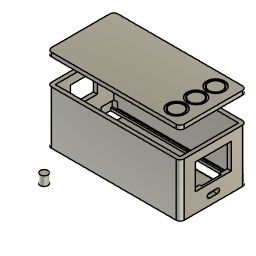
SmartClock v7 (Autodesk Fusion 360 design; units mm, degrees)
Autodesk Fusion 360 part; units mm, degrees
sketch "Sketch1" plane through (0, 0, 0) normal (0, 0, 1) x (1, 0, 0)
  line L0 (0, 0) -> (100, 0)
  line L1 (100, 0) -> (100, 50)
  line L2 (100, 50) -> (0, 50)
  line L3 (0, 50) -> (0, 0)
  line L4 (97, 47) -> (3, 47)
  line L5 (3, 47) -> (3, 3)
  line L6 (3, 3) -> (97, 3)
  line L7 (97, 3) -> (97, 47)
  dimension "boxOuterWidth" = 100
  dimension "boxOuterLength" = 50
  dimension "d3" = -3
  constraint horizontal L0
  constraint vertical L1
  constraint horizontal L2
  constraint vertical L3
  constraint coincident L0.start L3.end
  measures "boxOuterWidth" distance of L0.start L0.end
  measures "boxOuterLength" distance of L0.start L2.end
extrude "Extrude1" add sketch "Sketch1" along normal blind 3 contours L4 L5 L6 L7 makes body 1
extrude "Extrude2" add sketch "Sketch1" along normal blind 40 bodies 1
sketch "Sketch2" plane through (0, 0, 0) normal (-1, 0, 0) x (0, -1, 0)
  line L0 (-50, 0) -> (0, 0)
  line L1 (0, 0) -> (0, 40)
  line L2 (0, 40) -> (-50, 40)
  line L3 (-50, 40) -> (-50, 0)
  line L4 (-3, 3) -> (-47, 3)
  line L5 (-47, 3) -> (-47, 40)
  line L6 (-47, 40) -> (-3, 40)
  line L7 (-3, 40) -> (-3, 3)
  line L8 (-27.975, 12.2) -> (-22.025, 12.2)
  line L9 (-27.975, 8.7) -> (-22.025, 8.7)
  arc A0 (-22.025, 8.7) -> (-22.025, 12.2) centre (-22.025, 10.45) ccw
  arc A1 (-27.975, 12.2) -> (-27.975, 8.7) centre (-27.975, 10.45) ccw
  line L10 (-34.65, 34) -> (-34.65, 17.9)
  line L11 (-34.65, 17.9) -> (-14.35, 17.9)
  line L12 (-14.35, 17.9) -> (-14.35, 34)
  line L13 (-14.35, 34) -> (-34.65, 34)
  circle A2 centre (-12.1, 25.95) radius 1.4
  line L14 (-14.35, 25.95) -> (-34.65, 25.95) construction
  line L15 (-14.35, 25.95) -> (-12.1, 25.95) construction
  circle A3 centre (-12.1, 25.95) radius 2.25
  line L16 (-34.65, 25.95) -> (-39.95, 25.95) construction
  circle A4 centre (-39.95, 25.95) radius 1.45
  circle A5 centre (-39.95, 25.95) radius 2.5
  dimension "d8" = 5.95
  dimension "d9" = 3.5
  dimension "d10" = 16.1
  dimension "d11" = 20.3
  dimension "d12" = 2.8
  dimension "d13" = 2.25
  dimension "d19" = 5.3
  dimension "d20" = 2.9
  dimension "d21" = 5
  dimension "d25" = 12.35
  dimension "d26" = 6
  dimension "d27" = 5.7
  dimension "d28" = 5.7
  dimension "d29" = 19.025
  dimension "d30" = 19.025
  constraint horizontal L8
  constraint parallel L8 L9
  constraint tangent L9 A0
  constraint tangent L8 A0
  constraint tangent L9 A1
  constraint tangent L8 A1
  constraint midpoint L12 L14.start
  constraint midpoint L10 L14.end
  constraint perpendicular L12 L15
  constraint coincident A2.centre L15.end
  constraint concentric A2 A3
  constraint coincident L14.start A3
  constraint coincident L16.end A4.centre
  constraint perpendicular L10 L11
  constraint perpendicular L11 L12
  constraint perpendicular L12 L13
  constraint collinear L14 L16
  measures "d8" distance of L8.start L8.end
  measures "d9" distance of L8 L9
  measures "d10" distance of L10.start L10.end
  measures "d11" distance of L10.start L12.end
  measures "d12" diameter of A2
  measures "d13" distance of L12 A2.centre
  measures "d19" distance of L14.end L16.end
  measures "d20" diameter of A4
  measures "d21" diameter of A5
  measures "d25" distance of L5 L10
  measures "d26" distance of L2 L13
  measures "d27" distance of L4 L9
  measures "d28" distance of L8 L11
  measures "d29" distance of L5 A1.centre
  measures "d30" distance of L7 A0.centre
extrude "Extrude3" cut sketch "Sketch2" against normal up to surface (3 mm away) contours L8 L9 A0 A1 | L10 L11 L12 L13 bodies 1
extrude "Extrude4" add sketch "Sketch2" against normal blind 2 from surface at -3 contours A3 bodies 1
extrude "Extrude5" add sketch "Sketch2" against normal blind 4 from surface at -3 contours A5 bodies 1
sketch "Sketch3" plane through (100, 0, 0) normal (1, 0, 0) x (0, 1, 0)
  line L0 (0, 0) -> (50, 0)
  line L1 (50, 0) -> (50, 40)
  line L2 (50, 40) -> (0, 40)
  line L3 (0, 40) -> (0, 0)
  line L4 (47, 3) -> (3, 3)
  line L5 (3, 3) -> (3, 40)
  line L6 (3, 40) -> (47, 40)
  line L7 (47, 40) -> (47, 3)
  line L8 (22.025, 8.35) -> (27.975, 8.35)
  line L9 (22.025, 4.85) -> (27.975, 4.85)
  arc A0 (27.975, 4.85) -> (27.975, 8.35) centre (27.975, 6.6) ccw
  arc A1 (22.025, 8.35) -> (22.025, 4.85) centre (22.025, 6.6) ccw
  line L10 (19.5, 34.5) -> (30.5, 34.5)
  line L11 (13.25, 36) -> (36.75, 12.2) construction
  line L12 (38.55, 33.73) -> (38.55, 14.33)
  line L13 (13.25, 12.2) -> (13.25, 36) construction
  line L14 (36.75, 36) -> (36.75, 12.2) construction
  circle A2 centre (36.75, 36) radius 1.375
  line L15 (11.25, 33.73) -> (11.45, 33.73) construction
  line L16 (13.128, 19.766) -> (36.872, 19.766)
  line L17 (11.25, 38) -> (11.25, 33.73) construction
  line L18 (30.5, 38) -> (19.5, 38)
  line L19 (38.75, 32.63) -> (36.872, 32.63) construction
  line L20 (11.45, 33.73) -> (38.55, 33.73)
  line L21 (30.5, 34.5) -> (30.5, 38)
  line L22 (38.75, 38) -> (11.25, 38)
  circle A3 centre (36.75, 36) radius 0.975
  line L23 (19.5, 38) -> (19.5, 34.5)
  circle A4 centre (36.75, 12.2) radius 1.375
  circle A5 centre (13.25, 36) radius 0.975
  line L24 (17.5, 10.2) -> (17.5, 14.2)
  line L25 (13.128, 32.63) -> (13.128, 19.766)
  circle A6 centre (13.25, 36) radius 1.375
  line L26 (11.45, 14.33) -> (11.45, 33.73)
  line L27 (32.5, 14.2) -> (32.5, 14.33)
  line L28 (36.872, 32.63) -> (13.128, 32.63)
  line L29 (32.5, 10.2) -> (17.5, 14.2) construction
  line L30 (36.872, 19.766) -> (36.872, 32.63)
  circle A7 centre (13.25, 12.2) radius 0.975
  line L31 (38.75, 38) -> (38.75, 32.63) construction
  line L32 (13.25, 36) -> (36.75, 36) construction
  line L33 (38.55, 14.33) -> (11.45, 14.33)
  circle A8 centre (36.75, 12.2) radius 0.975
  line L34 (32.5, 10.2) -> (17.5, 10.2)
  circle A9 centre (13.25, 12.2) radius 1.375
  line L35 (17.5, 10.2) -> (32.5, 14.2) construction
  line L36 (17.5, 14.2) -> (17.5, 14.33)
  line L37 (36.75, 12.2) -> (13.25, 12.2) construction
  line L38 (17.5, 14.2) -> (32.5, 14.2)
  line L39 (11.25, 10.2) -> (38.75, 10.2)
  line L40 (32.5, 14.2) -> (32.5, 10.2)
  line L41 (38.75, 10.2) -> (38.75, 38)
  line L42 (11.25, 38) -> (38.75, 10.2) construction
  line L43 (11.25, 38) -> (11.25, 10.2)
  line L44 (25, 38) -> (30.5, 38) construction
  line L45 (38.75, 38) -> (11.25, 10.2) construction
  line L46 (36.75, 36) -> (13.25, 12.2) construction
  line L47 (25, 40) -> (25, 3) construction
  line L48 (17.5, 14.2) -> (17.5, 14.33)
  line L49 (32.5, 14.2) -> (32.5, 14.33)
  point P0 (25, 12.2)
  point P1 (25, 24.1)
  point P2 (25, 24.1)
  dimension "d31" = 3.5
  dimension "d32" = 5.95
  dimension "d33" = 27.5
  dimension "d34" = 27.8
  dimension "d35" = 23.5
  dimension "d36" = 23.8
  dimension "d37" = 1.95
  dimension "d38" = 1.95
  dimension "d39" = 1.95
  dimension "d40" = 1.95
  dimension "d41" = 5.37
  dimension "d42" = 1.878
  dimension "d43" = 23.744
  dimension "d44" = 12.864
  dimension "d45" = 4.27
  dimension "d46" = 0.2
  dimension "d47" = 27.1
  dimension "d48" = 19.4
  dimension "d49" = 5.5
  dimension "d50" = 11
  dimension "d51" = 3.5
  dimension "d52" = 15
  dimension "d53" = 2.75
  dimension "d54" = 2.75
  dimension "d55" = 2.75
  dimension "d56" = 2.75
  dimension "d57" = 19.025
  dimension "d58" = 19.025
  dimension "d59" = 2
  dimension "d60" = 1.85
  dimension "d61" = 1.85
  constraint perpendicular L3 L8
  constraint parallel L8 L9
  constraint tangent L9 A0
  constraint tangent L8 A0
  constraint tangent L9 A1
  constraint tangent L8 A1
  constraint horizontal L22
  constraint perpendicular L22 L43
  constraint parallel L22 L39
  constraint parallel L41 L43
  constraint coincident P2 L45
  constraint coincident P2 L42
  constraint horizontal L32
  constraint perpendicular L14 L32
  constraint parallel L32 L37
  constraint parallel L13 L14
  constraint coincident P2 L11
  constraint coincident P2 L46
  constraint coincident P2 P1
  constraint coincident L11.start L13.end
  constraint perpendicular L22 L31
  constraint perpendicular L19 L31
  constraint horizontal L28
  constraint vertical L25
  constraint horizontal L16
  constraint vertical L30
  constraint perpendicular L17 L22
  constraint perpendicular L15 L17
  constraint horizontal L20
  constraint vertical L12
  constraint horizontal L33
  constraint vertical L26
  constraint midpoint L44.start L22
  constraint horizontal L18
  constraint vertical L23
  constraint horizontal L10
  constraint vertical L21
  constraint horizontal L34
  constraint perpendicular L24 L34
  constraint parallel L34 L38
  constraint parallel L24 L40
  constraint coincident P0 L29
  constraint coincident P0 L35
  constraint coincident L29.start L39
  constraint midpoint P0 L37
  constraint coincident L36.end L33
  constraint perpendicular L33 L36
  constraint coincident L27.end L33
  constraint perpendicular L27 L33
  constraint concentric A2 A3
  constraint concentric A4 A8
  constraint concentric A7 A9
  constraint concentric A5 A6
  constraint midpoint L6 L47.start
  constraint midpoint L4 L47.end
  constraint coincident P2 L47
  constraint coincident L18.start L22
  constraint coincident L14.start A2.centre
  constraint coincident L11.end L14.end
  constraint coincident L13.start A7.centre
  measures "d31" distance of L8 L9
  measures "d32" distance of L8.start L8.end
  measures "d33" distance of L39.start L39.end
  measures "d34" distance of L39.start L17.start
  measures "d35" distance of L11.end L13.start
  measures "d36" distance of L11.end L14.start
  measures "d37" diameter of A5
  measures "d38" diameter of A7
  measures "d39" diameter of A8
  measures "d40" diameter of A3
  measures "d41" distance of L22.start L19.start
  measures "d42" distance of L19.start L19.end
  measures "d43" distance of L25.start L19.end
  measures "d44" distance of L19.end L16.end
  measures "d45" distance of L15.start L17.start
  measures "d46" distance of L15.start L15.end
  measures "d47" distance of L12.start L15.end
  measures "d48" distance of L26.start L15.end
  measures "d49" distance of L18.start L44.start
  measures "d50" distance of L18.start L18.end
  measures "d51" distance of L18.start L10.end
  measures "d52" distance of L27.start L24.end
  measures "d53" diameter of A2
  measures "d54" diameter of A4
  measures "d55" diameter of A9
  measures "d56" diameter of A6
  measures "d57" distance of L5 A1.centre
  measures "d58" distance of L7 A0.centre
  measures "d59" distance of L2 L22
  measures "d60" distance of L8 L39
  measures "d61" distance of L4 L9
extrude "Extrude6" cut sketch "Sketch3" against normal up to surface (3 mm away) contours L8 L9 A0 A1 | L12 L20 L26 L33 | L16 L25 L28 L30 bodies 1
extrude "Extrude7" cut sketch "Sketch3" along normal blind 2 from surface at -3 contours A3 | A5 | A7 | A8 bodies 1
extrude "Extrude8" add sketch "Sketch3" against normal blind 0.5 from surface at -3 contours A2 | A4 | A6 | A9 bodies 1
extrude "Extrude9" cut sketch "Sketch3" along normal blind 1.5 from surface at -3 contours L24 L34 L38 L39 L40 | L27 L33 L36 L38 L48 L49 bodies 1
fillet "Fillet1" radius 3 4 edges at (0, 0, 20) (0, 50, 20) (100, 50, 20) (100, 0, 20) on bodies 1
extrude "Extrude10" add 1 faces at (34.3333, 17.6667, 3) along direction (0, 0, 1) blind 3 from surface at 37 separate body on bodies 1 makes body 2
extrude "Extrude11" add 1 faces at (65.6667, 1, 40) along direction (0, 0, 1) blind 3 separate body on bodies 1 makes body 3
move_body "Move1" bodies 2 3 to x (1, 0, 0) y (0, 1, 0) z (0, 0, 1) at (0, 0, 19.6311)
extrude "Extrude12" add 1 faces at (34.3333, 17.6667, 59.6311) along direction (0, 0, -1) blind 2 on bodies 2 bodies 2 3
sketch "Sketch4" plane through (0, 0, 57.6311) normal (0, 0, -1) x (1, 0, 0)
  line L0 (97, -3) -> (3, -3)
  line L1 (3, -3) -> (3, -47)
  line L2 (3, -47) -> (97, -47)
  line L3 (97, -47) -> (97, -3)
  line L4 (87, -3) -> (87, -47) construction
  circle A0 centre (87, -39.6667) radius 5
  circle A1 centre (87, -25) radius 5
  circle A2 centre (87, -10.3333) radius 5
  circle A3 centre (87, -10.3333) radius 6.75
  circle A4 centre (87, -25) radius 6.75
  circle A5 centre (87, -39.6667) radius 6.75
  circle A6 centre (87, -39.6667) radius 5.5
  circle A7 centre (87, -25) radius 5.5
  circle A8 centre (87, -10.3333) radius 5.5
  dimension "d82" = 10
  dimension "d83" = 10
  dimension "d84" = 10
  dimension "d85" = 10
  dimension "d86" = 7.3333
  dimension "d87" = 14.6667
  dimension "d88" = 14.6667
  dimension "d90" = 7.3333
  dimension "d91" = 1.75
  dimension "d92" = 1.75
  dimension "d93" = 1.75
  dimension "d99" = 0.5
  dimension "d100" = 0.5
  dimension "d101" = 0.5
  constraint coincident L0 L4.start
  constraint coincident L2 L4.end
  constraint perpendicular L2 L4
  constraint coincident L4 A0.centre
  constraint coincident L4 A1.centre
  constraint coincident L4 A2.centre
  measures "d82" distance of L3 L4
  measures "d83" diameter of A0
  measures "d84" diameter of A1
  measures "d85" diameter of A2
  measures "d86" distance of L2 A0.centre
  measures "d87" distance of A0.centre A1.centre
  measures "d88" distance of A1.centre A2.centre
  measures "d90" distance of L0 A2.centre
extrude "Extrude13" cut sketch "Sketch4" against normal blind 4.6 contours A0 | A1 | A2 bodies 2
extrude "Extrude14" cut sketch "Sketch4" along normal blind 0.5 from surface at -5 contours A3 | A4 | A5 bodies 2
sketch "Sketch5" plane through (0, 0, 0) normal (0, 0, -1) x (1, 0, 0)
  arc A0 (100, -3) -> (97, 0) centre (97, -3) ccw
  line L0 (0, -3) -> (0, -47)
  arc A1 (0, -47) -> (3, -50) centre (3, -47) ccw
  line L1 (3, -50) -> (97, -50)
  arc A2 (97, -50) -> (100, -47) centre (97, -47) ccw
  line L2 (100, -47) -> (100, -3)
  line L3 (0.8, -2) -> (99.2, -2)
  line L4 (99.2, -2) -> (99.2, -12.5)
  line L5 (99.2, -12.5) -> (0.8, -12.5)
  line L6 (0.8, -12.5) -> (0.8, -2)
  arc A3 (100, -3) -> (97, 0) centre (97, -3) ccw
  line L7 (99.2, -48) -> (0.8, -48)
  line L8 (0.8, -48) -> (0.8, -37.5)
  line L9 (0.8, -37.5) -> (99.2, -37.5)
  line L10 (99.2, -37.5) -> (99.2, -48)
  line L11 (3, 0) -> (97, 0)
  line L12 (99.2, -42.75) -> (0.8, -42.75) construction
  line L13 (0.8, -46.75) -> (99.2, -46.75)
  line L14 (99.2, -46.75) -> (99.2, -38.75)
  line L15 (99.2, -38.75) -> (0.8, -38.75)
  line L16 (0.8, -38.75) -> (0.8, -46.75)
  line L17 (0.8, -46.75) -> (99.2, -38.75) construction
  line L18 (99.2, -46.75) -> (0.8, -38.75) construction
  line L19 (0.8, -7.25) -> (99.2, -7.25) construction
  line L20 (99.2, -3.25) -> (0.8, -3.25)
  line L21 (0.8, -3.25) -> (0.8, -11.25)
  line L22 (0.8, -11.25) -> (99.2, -11.25)
  line L23 (99.2, -11.25) -> (99.2, -3.25)
  line L24 (99.2, -3.25) -> (0.8, -11.25) construction
  line L25 (0.8, -3.25) -> (99.2, -11.25) construction
  line L26 (5.8, -48) -> (5.8, -2)
  line L27 (94.2, -2) -> (94.2, -48)
  circle A4 centre (8.8, -15.5) radius 3
  circle A5 centre (91.2, -15.5) radius 3
  circle A6 centre (91.2, -34.5) radius 3
  circle A7 centre (8.8, -34.5) radius 3
  point P0 (50, -42.75)
  point P1 (50, -7.25)
  dimension "d102" = 98.4
  dimension "d103" = 10.5
  dimension "d106" = 98.4
  dimension "d107" = 10.5
  dimension "d111" = 2
  dimension "d112" = 0.8
  dimension "d113" = 0.8
  dimension "d114" = 2
  dimension "d115" = 0.8
  dimension "d124" = 8
  dimension "d127" = 8
  dimension "d128" = 5
  dimension "d132" = 5
  dimension "d133" = 3
  dimension "d134" = 3
  dimension "d135" = 3
  dimension "d136" = 3
  constraint horizontal L3
  constraint vertical L4
  constraint horizontal L5
  constraint vertical L6
  constraint horizontal L9
  constraint vertical L10
  constraint horizontal L7
  constraint vertical L8
  constraint midpoint L10 L12.start
  constraint midpoint L8 L12.end
  constraint horizontal L13
  constraint perpendicular L13 L14
  constraint parallel L13 L15
  constraint parallel L14 L16
  constraint coincident L17 P0
  constraint coincident L18 P0
  constraint coincident L8 L13.start
  constraint midpoint L12 P0
  constraint midpoint L6 L19.start
  constraint midpoint L4 L19.end
  constraint horizontal L20
  constraint perpendicular L20 L21
  constraint parallel L20 L22
  constraint parallel L21 L23
  constraint coincident L24 P1
  constraint coincident L25 P1
  constraint coincident L4 L20.start
  constraint midpoint L19 P1
  constraint coincident L7 L26.start
  constraint coincident L3 L26.end
  constraint perpendicular L3 L26
  constraint coincident L3 L27.start
  constraint coincident L7 L27.end
  constraint perpendicular L7 L27
  constraint tangent L5 A4
  constraint tangent L26 A4
  constraint tangent L5 A5
  constraint tangent L27 A5
  constraint tangent L9 A6
  constraint tangent L27 A6
  constraint tangent L26 A7
  constraint tangent L9 A7
  measures "d102" distance of L3.start L3.end
  measures "d103" distance of L3.start L5.end
  measures "d106" distance of L9.end L8.end
  measures "d107" distance of L7.end L8.end
  measures "d111" distance of L3 L11
  measures "d112" distance of L0 L6
  measures "d113" distance of L2 L4
  measures "d114" distance of L1 L7
  measures "d115" distance of L0 L8
  measures "d124" distance of L13.end L14.end
  measures "d127" distance of L20.end L21.end
  measures "d128" distance of L8 L26
  measures "d132" distance of L10 L27
  measures "d133" radius of A4
  measures "d134" radius of A5
  measures "d135" radius of A6
  measures "d136" radius of A7
extrude "Extrude15" cut sketch "Sketch5" along normal blind 1 and the other way blind 1 from surface at -3 contours L3 L6 L20 L26 | L3 L20 L26 L27 | L6 L20 L21 L22 L26 | L3 L4 L20 L27 | L20 L22 L26 L27 | L5 L6 L22 L26 | L4 L20 L22 L23 L27 | L5 L22 L26 L27 | L4 L5 L22 L27 | L8 L9 L15 L26 | L9 L15 L26 L27 | L9 L10 L15 L27 | L8 L13 L15 L16 L26 | L13 L15 L26 L27 | L10 L13 L14 L15 L27 | L7 L8 L13 L26 | L7 L13 L26 L27 | L7 L10 L13 L27 bodies 1
extrude "Extrude16" cut sketch "Sketch5" against normal up to surface (2 mm away) contours L6 L20 L21 L22 L26 | L20 L22 L26 L27 | L4 L20 L22 L23 L27 | L8 L13 L15 L16 L26 | L13 L15 L26 L27 | L10 L13 L14 L15 L27 bodies 1
extrude "Extrude17" cut sketch "Sketch5" against normal blind 5 from surface at -3 contours L3 L6 L20 L26 | L6 L20 L21 L22 L26 | L3 L4 L20 L27 | L5 L6 L22 L26 | L4 L20 L22 L23 L27 | L4 L5 L22 L27 | L8 L9 L15 L26 | L9 L10 L15 L27 | L8 L13 L15 L16 L26 | L10 L13 L14 L15 L27 | L7 L8 L13 L26 | L7 L10 L13 L27 bodies 1
extrude "Extrude18" cut sketch "Sketch5" against normal blind 2 contours A4 | A5 | A7 | A6 bodies 1
cylinder "CylinderPrimitive1" add diameter 5.75 height 7 placed x (1, 0, 0) y (0, 1, 0) z (0, 0, 1) at (23.2634, -25.7219, 0) separate body makes body 4
sketch "Sketch8" plane through (0, 0, 3) normal (0, 0, 1) x (-1, 0, 0)
  line L0 (-3, -12.5) -> (-97, -12.5)
  line L1 (-97, -12.5) -> (-97, -37.5)
  line L2 (-97, -37.5) -> (-3, -37.5)
  line L3 (-3, -37.5) -> (-3, -12.5)
  line L4 (-3, -25) -> (-97, -25) construction
  line L5 (-50, -37.5) -> (-50, -12.5) construction
  line L6 (-22.5, -16) -> (-77.5, -16)
  line L7 (-77.5, -16) -> (-77.5, -34)
  line L8 (-77.5, -34) -> (-22.5, -34)
  line L9 (-22.5, -34) -> (-22.5, -16)
  line L10 (-22.5, -16) -> (-77.5, -34) construction
  line L11 (-77.5, -16) -> (-22.5, -34) construction
  point P0 (-50, -25)
  dimension "d141" = 55
  dimension "d142" = 18
  constraint midpoint L3 L4.start
  constraint midpoint L1 L4.end
  constraint midpoint L2 L5.start
  constraint midpoint L0 L5.end
  constraint horizontal L6
  constraint perpendicular L6 L7
  constraint parallel L6 L8
  constraint parallel L7 L9
  constraint coincident L10 P0
  constraint coincident L11 P0
  constraint coincident L5 P0
  constraint coincident L4 P0
  measures "d141" distance of L6.start L6.end
  measures "d142" distance of L6.start L8.end
extrude "Extrude19" add sketch "Sketch8" along normal blind 10 contours L6 L7 L8 L9 bodies 1
equation "boxOuterHeight = 40 mm"
equation "d8 = 9.1 mm - 3.15 mm"
equation "d25 = ( 45 mm - d11 ) / 2"
equation "d27 = d28"
equation "d29 = d30"
equation "d32 = 9.1 mm - 3.15 mm"
equation "d57 = d58"
equation "d60 = d61"
equation "d86 = d90"
equation "d87 = ( 44 / 3 ) * 1 mm"
equation "d88 = d87"
equation "d102 = d106"
equation "d106 = 100 mm - 1.6 mm"
equation "d112 = d113"
equation "d139 = 2 mm + 5 mm"
named bodies: "Body", "Cap", "Foot"
